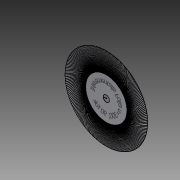
# Autodesk Inventor part: InkrementalisFolia
Saved by Autodesk Inventor 2015 (Build 190159000, 159)
## iProperties
Created: 2014-11-14
Part Number: InkrementalisFolia
Material: Generic
Document SubType Name: Modeling
Designer: laca
Density: 1 g/cm^3
Appearance: Default
Mass: 0.167133 g
Surface Area: 16.952 cm^2
Volume: 0.167133 cm^3
d32: 360.00 deg
Author: laca
Autodesk Inventor part; units mm, degrees
ref_plane "YZ Plane" through (0, 0, 0) normal (1, 0, 0) x (0, 1, 0)
ref_plane "XZ Plane" through (0, 0, 0) normal (0, 1, 0) x (-1, 0, 0)
ref_plane "XY Plane" through (0, 0, 0) normal (0, 0, 1) x (1, 0, 0)
sketch "Sketch1" plane through (0, 0, 0) normal (0, 1, 0) x (-1, 0, 0)
  circle A0 centre (0, 0) radius 32.5
  circle A1 centre (0, 0) radius 22.5
  circle A2 centre (0, 0) radius 16
  line L0 (22.5, 0) -> (32.5, 0)
  line L1 (22.4991, -0.1963) -> (32.4988, -0.2836)
  dimension "d0" = 65
  dimension "d2" = 10
  dimension "d3" = 32
  dimension "d12" = 0.5
  constraints: 4 end point, 4 point on circle, 3 centre point, 3 coincident, 1 horizontal
  measures "d0" diameter of A0
  measures "d2" radial gap between concentric circles of A0 A1
  measures "d3" diameter of A2
  measures "d12" angle of L1 L0
extrude "Extrusion1" [suppressed]
extrude "Extrusion2" [suppressed]
pattern_circular "Circular Pattern1" [suppressed]
sketch "Sketch3" plane through (0, 0, 0) normal (0, 0, 1) x (1, 0, 0)
  circle A0 centre (0, 0) radius 33
  circle A1 centre (0, 0) radius 16.5
  circle A2 centre (0, 0) radius 2.5
  line L0 (-16.2493, -2.8652) -> (-16.2493, -28.7221)
  line L1 (0, 0) -> (-2.5, 0)
  line L2 (-16.1394, -3.4305) -> (-15.237, -29.2717)
  line L3 (-16.0099, -3.9917) -> (-14.2062, -29.7856)
  line L4 (-15.8608, -4.548) -> (-13.158, -30.2633)
  line L5 (-15.6924, -5.0988) -> (-12.0938, -30.7041)
  line L6 (-15.5049, -5.6433) -> (-11.0149, -31.1074)
  line L7 (-15.2985, -6.181) -> (-9.9226, -31.4729)
  line L8 (-15.0735, -6.7112) -> (-8.8181, -31.8)
  line L9 (-14.8301, -7.2331) -> (-7.703, -32.0884)
  line L10 (-14.5686, -7.7463) -> (-6.5784, -32.3377)
  line L11 (-14.2894, -8.25) -> (-5.4458, -32.5475)
  line L12 (-13.9928, -8.7437) -> (-4.3066, -32.7178)
  line L13 (-13.6791, -9.2267) -> (-3.1622, -32.8481)
  line L14 (-13.3488, -9.6985) -> (-2.0139, -32.9385)
  line L15 (-13.0022, -10.1584) -> (-0.8631, -32.9887)
  line L16 (-12.6397, -10.606) -> (0.2887, -32.9987)
  line L17 (-12.2619, -11.0407) -> (1.4402, -32.9686)
  line L18 (-11.8691, -11.4619) -> (2.5899, -32.8982)
  line L19 (-11.4619, -11.8691) -> (3.7364, -32.7878)
  line L20 (-11.0407, -12.2619) -> (4.8784, -32.6374)
  line L21 (-10.606, -12.6397) -> (6.0145, -32.4473)
  line L22 (-10.1584, -13.0022) -> (7.1432, -32.2176)
  line L23 (-9.6985, -13.3488) -> (8.2633, -31.9487)
  line L24 (-9.2267, -13.6791) -> (9.3732, -31.6408)
  line L25 (-8.7437, -13.9928) -> (10.4718, -31.2944)
  line L26 (-8.25, -14.2894) -> (11.5575, -30.9099)
  line L27 (-7.7463, -14.5686) -> (12.6292, -30.4877)
  line L28 (-7.2331, -14.8301) -> (13.6856, -30.0284)
  line L29 (-6.7112, -15.0735) -> (14.7252, -29.5325)
  line L30 (-6.181, -15.2985) -> (15.7469, -29.0006)
  line L31 (-5.6433, -15.5049) -> (16.7494, -28.4334)
  line L32 (-5.0988, -15.6924) -> (17.7315, -27.8315)
  line L33 (-4.548, -15.8608) -> (18.692, -27.1957)
  line L34 (-3.9917, -16.0099) -> (19.6298, -26.5268)
  line L35 (-3.4305, -16.1394) -> (20.5436, -25.8256)
  line L36 (-2.8652, -16.2493) -> (21.4324, -25.0929)
  line L37 (-2.2964, -16.3394) -> (22.295, -24.3296)
  line L38 (-1.7247, -16.4096) -> (23.1305, -23.5367)
  line L39 (-1.151, -16.4598) -> (23.9379, -22.7152)
  line L40 (-0.5758, -16.4899) -> (24.716, -21.8659)
  line L41 (0, -16.5) -> (25.4641, -20.99)
  line L42 (0.5758, -16.4899) -> (26.1811, -20.0885)
  line L43 (1.151, -16.4598) -> (26.8662, -19.1626)
  line L44 (1.7247, -16.4096) -> (27.5186, -18.2133)
  line L45 (2.2964, -16.3394) -> (28.1375, -17.2418)
  line L46 (2.8652, -16.2493) -> (28.7221, -16.2493)
  line L47 (3.4305, -16.1394) -> (29.2717, -15.237)
  line L48 (3.9917, -16.0099) -> (29.7856, -14.2062)
  line L49 (4.548, -15.8608) -> (30.2633, -13.158)
  line L50 (5.0988, -15.6924) -> (30.7041, -12.0938)
  line L51 (5.6433, -15.5049) -> (31.1074, -11.0149)
  line L52 (6.181, -15.2985) -> (31.4729, -9.9226)
  line L53 (6.7112, -15.0735) -> (31.8, -8.8181)
  line L54 (7.2331, -14.8301) -> (32.0884, -7.703)
  line L55 (7.7463, -14.5686) -> (32.3377, -6.5784)
  line L56 (8.25, -14.2894) -> (32.5475, -5.4458)
  line L57 (8.7437, -13.9928) -> (32.7178, -4.3066)
  line L58 (9.2267, -13.6791) -> (32.8481, -3.1622)
  line L59 (9.6985, -13.3488) -> (32.9385, -2.0139)
  line L60 (10.1584, -13.0022) -> (32.9887, -0.8631)
  line L61 (10.606, -12.6397) -> (32.9987, 0.2887)
  line L62 (11.0407, -12.2619) -> (32.9686, 1.4402)
  line L63 (11.4619, -11.8691) -> (32.8982, 2.5899)
  line L64 (11.8691, -11.4619) -> (32.7878, 3.7364)
  line L65 (12.2619, -11.0407) -> (32.6374, 4.8784)
  line L66 (12.6397, -10.606) -> (32.4473, 6.0145)
  line L67 (13.0022, -10.1584) -> (32.2176, 7.1432)
  line L68 (13.3488, -9.6985) -> (31.9487, 8.2633)
  line L69 (13.6791, -9.2267) -> (31.6408, 9.3732)
  line L70 (13.9928, -8.7437) -> (31.2944, 10.4718)
  line L71 (14.2894, -8.25) -> (30.9099, 11.5575)
  line L72 (14.5686, -7.7463) -> (30.4877, 12.6292)
  line L73 (14.8301, -7.2331) -> (30.0284, 13.6856)
  line L74 (15.0735, -6.7112) -> (29.5325, 14.7252)
  line L75 (15.2985, -6.181) -> (29.0006, 15.7469)
  line L76 (15.5049, -5.6433) -> (28.4334, 16.7494)
  line L77 (15.6924, -5.0988) -> (27.8315, 17.7315)
  line L78 (15.8608, -4.548) -> (27.1957, 18.692)
  line L79 (16.0099, -3.9917) -> (26.5268, 19.6298)
  line L80 (16.1394, -3.4305) -> (25.8256, 20.5436)
  line L81 (16.2493, -2.8652) -> (25.0929, 21.4324)
  line L82 (16.3394, -2.2964) -> (24.3296, 22.295)
  line L83 (16.4096, -1.7247) -> (23.5367, 23.1305)
  line L84 (16.4598, -1.151) -> (22.7152, 23.9379)
  line L85 (16.4899, -0.5758) -> (21.8659, 24.716)
  line L86 (16.5, 0) -> (20.99, 25.4641)
  line L87 (16.4899, 0.5758) -> (20.0885, 26.1811)
  line L88 (16.4598, 1.151) -> (19.1626, 26.8662)
  line L89 (16.4096, 1.7247) -> (18.2133, 27.5186)
  line L90 (16.3394, 2.2964) -> (17.2418, 28.1375)
  line L91 (16.2493, 2.8652) -> (16.2493, 28.7221)
  line L92 (16.1394, 3.4305) -> (15.237, 29.2717)
  line L93 (16.0099, 3.9917) -> (14.2062, 29.7856)
  line L94 (15.8608, 4.548) -> (13.158, 30.2633)
  line L95 (15.6924, 5.0988) -> (12.0938, 30.7041)
  line L96 (15.5049, 5.6433) -> (11.0149, 31.1074)
  line L97 (15.2985, 6.181) -> (9.9226, 31.4729)
  line L98 (15.0735, 6.7112) -> (8.8181, 31.8)
  line L99 (14.8301, 7.2331) -> (7.703, 32.0884)
  line L100 (14.5686, 7.7463) -> (6.5784, 32.3377)
  line L101 (14.2894, 8.25) -> (5.4458, 32.5475)
  line L102 (13.9928, 8.7437) -> (4.3066, 32.7178)
  line L103 (13.6791, 9.2267) -> (3.1622, 32.8481)
  line L104 (13.3488, 9.6985) -> (2.0139, 32.9385)
  line L105 (13.0022, 10.1584) -> (0.8631, 32.9887)
  line L106 (12.6397, 10.606) -> (-0.2887, 32.9987)
  line L107 (12.2619, 11.0407) -> (-1.4402, 32.9686)
  line L108 (11.8691, 11.4619) -> (-2.5899, 32.8982)
  line L109 (11.4619, 11.8691) -> (-3.7364, 32.7878)
  line L110 (11.0407, 12.2619) -> (-4.8784, 32.6374)
  line L111 (10.606, 12.6397) -> (-6.0145, 32.4473)
  line L112 (10.1584, 13.0022) -> (-7.1432, 32.2176)
  line L113 (9.6985, 13.3488) -> (-8.2633, 31.9487)
  line L114 (9.2267, 13.6791) -> (-9.3732, 31.6408)
  line L115 (8.7437, 13.9928) -> (-10.4718, 31.2944)
  line L116 (8.25, 14.2894) -> (-11.5575, 30.9099)
  line L117 (7.7463, 14.5686) -> (-12.6292, 30.4877)
  line L118 (7.2331, 14.8301) -> (-13.6856, 30.0284)
  line L119 (6.7112, 15.0735) -> (-14.7252, 29.5325)
  line L120 (6.181, 15.2985) -> (-15.7469, 29.0006)
  line L121 (5.6433, 15.5049) -> (-16.7494, 28.4334)
  line L122 (5.0988, 15.6924) -> (-17.7315, 27.8315)
  line L123 (4.548, 15.8608) -> (-18.692, 27.1957)
  line L124 (3.9917, 16.0099) -> (-19.6298, 26.5268)
  line L125 (3.4305, 16.1394) -> (-20.5436, 25.8256)
  line L126 (2.8652, 16.2493) -> (-21.4324, 25.0929)
  line L127 (2.2964, 16.3394) -> (-22.295, 24.3296)
  line L128 (1.7247, 16.4096) -> (-23.1305, 23.5367)
  line L129 (1.151, 16.4598) -> (-23.9379, 22.7152)
  line L130 (0.5758, 16.4899) -> (-24.716, 21.8659)
  line L131 (0, 16.5) -> (-25.4641, 20.99)
  line L132 (-0.5758, 16.4899) -> (-26.1811, 20.0885)
  line L133 (-1.151, 16.4598) -> (-26.8662, 19.1626)
  line L134 (-1.7247, 16.4096) -> (-27.5186, 18.2133)
  line L135 (-2.2964, 16.3394) -> (-28.1375, 17.2418)
  line L136 (-2.8652, 16.2493) -> (-28.7221, 16.2493)
  line L137 (-3.4305, 16.1394) -> (-29.2717, 15.237)
  line L138 (-3.9917, 16.0099) -> (-29.7856, 14.2062)
  line L139 (-4.548, 15.8608) -> (-30.2633, 13.158)
  line L140 (-5.0988, 15.6924) -> (-30.7041, 12.0938)
  line L141 (-5.6433, 15.5049) -> (-31.1074, 11.0149)
  line L142 (-6.181, 15.2985) -> (-31.4729, 9.9226)
  line L143 (-6.7112, 15.0735) -> (-31.8, 8.8181)
  line L144 (-7.2331, 14.8301) -> (-32.0884, 7.703)
  line L145 (-7.7463, 14.5686) -> (-32.3377, 6.5784)
  line L146 (-8.25, 14.2894) -> (-32.5475, 5.4458)
  line L147 (-8.7437, 13.9928) -> (-32.7178, 4.3066)
  line L148 (-9.2267, 13.6791) -> (-32.8481, 3.1622)
  line L149 (-9.6985, 13.3488) -> (-32.9385, 2.0139)
  line L150 (-10.1584, 13.0022) -> (-32.9887, 0.8631)
  line L151 (-10.606, 12.6397) -> (-32.9987, -0.2887)
  line L152 (-11.0407, 12.2619) -> (-32.9686, -1.4402)
  line L153 (-11.4619, 11.8691) -> (-32.8982, -2.5899)
  line L154 (-11.8691, 11.4619) -> (-32.7878, -3.7364)
  line L155 (-12.2619, 11.0407) -> (-32.6374, -4.8784)
  line L156 (-12.6397, 10.606) -> (-32.4473, -6.0145)
  line L157 (-13.0022, 10.1584) -> (-32.2176, -7.1432)
  line L158 (-13.3488, 9.6985) -> (-31.9487, -8.2633)
  line L159 (-13.6791, 9.2267) -> (-31.6408, -9.3732)
  line L160 (-13.9928, 8.7437) -> (-31.2944, -10.4718)
  line L161 (-14.2894, 8.25) -> (-30.9099, -11.5575)
  line L162 (-14.5686, 7.7463) -> (-30.4877, -12.6292)
  line L163 (-14.8301, 7.2331) -> (-30.0284, -13.6856)
  line L164 (-15.0735, 6.7112) -> (-29.5325, -14.7252)
  line L165 (-15.2985, 6.181) -> (-29.0006, -15.7469)
  line L166 (-15.5049, 5.6433) -> (-28.4334, -16.7494)
  line L167 (-15.6924, 5.0988) -> (-27.8315, -17.7315)
  line L168 (-15.8608, 4.548) -> (-27.1957, -18.692)
  line L169 (-16.0099, 3.9917) -> (-26.5268, -19.6298)
  line L170 (-16.1394, 3.4305) -> (-25.8256, -20.5436)
  line L171 (-16.2493, 2.8652) -> (-25.0929, -21.4324)
  line L172 (-16.3394, 2.2964) -> (-24.3296, -22.295)
  line L173 (-16.4096, 1.7247) -> (-23.5367, -23.1305)
  line L174 (-16.4598, 1.151) -> (-22.7152, -23.9379)
  line L175 (-16.4899, 0.5758) -> (-21.8659, -24.716)
  line L176 (-16.5, 0) -> (-20.99, -25.4641)
  line L177 (-16.4899, -0.5758) -> (-20.0885, -26.1811)
  line L178 (-16.4598, -1.151) -> (-19.1626, -26.8662)
  line L179 (-16.4096, -1.7247) -> (-18.2133, -27.5186)
  line L180 (-16.3394, -2.2964) -> (-17.2418, -28.1375)
  dimension "d21" = 66
  dimension "d27" = 33
  dimension "d28" = 5
  dimension "d29" = 90
  dimension "d32" = 360
  constraints: 362 end point, 3 coincident, 1 horizontal, 1 horizontal alignment, 549 other
  measures "d29" angle of L0 L1
extrude "Extrusion6" add sketch "Sketch3" along normal blind 0.1
body "Solid1"
